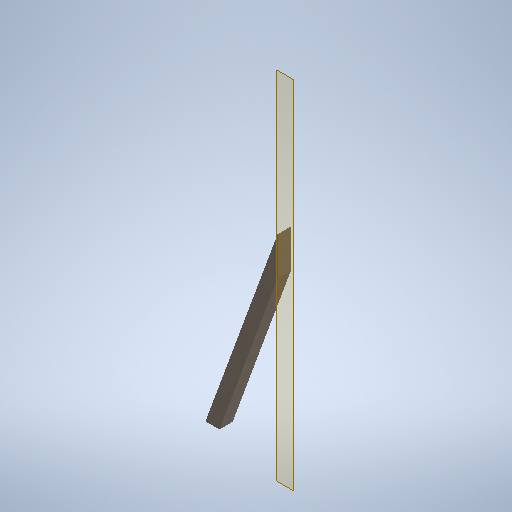
# Autodesk Inventor part: BaseAngularLarge
Saved by Autodesk Inventor 2025.2 (Build 292293000, 293)
## iProperties
Created: 2025-03-06
Part Number: BaseAngularLarge
Material: Wood (Walnut)
Document SubType Name: Modeling
Designer: baolo
Density: 0.55 g/cm^3
Appearance: Walnut
Mass: 84.4562 g
Surface Area: 320.992 cm^2
Volume: 153.557 cm^3
Author: baolo
Autodesk Inventor part; units mm, degrees
ref_plane "YZ Plane" through (0, 0, 0) normal (1, 0, 0) x (0, 1, 0)
ref_plane "XZ Plane" through (0, 0, 0) normal (0, 1, 0) x (-1, 0, 0)
ref_plane "XY Plane" through (0, 0, 0) normal (0, 0, 1) x (1, 0, 0)
ref_plane "Work Plane1" through (0, 0, 0) normal (0, 0, 1) x (1, 0, 0)
sketch "Sketch1" plane through (0, 0, 0) normal (0, 0, 1) x (1, 0, 0)
  line L0 (-95.7656, 0) -> (-77.1824, 0)
  line L1 (-77.1824, 0) -> (0, 212.057)
  line L2 (0, 212.057) -> (0, 263.1139)
  line L3 (0, 263.1139) -> (-95.7656, 0)
  line L4 (-205, 0) -> (-205, -20) construction
  line L5 (0, 0) -> (0, 430) construction
  line L6 (-205, 0) -> (225, 0) construction
  line L7 (-55.0006, 112.001) -> (-38.5912, 106.0285) construction
  line L8 (0, 263.1139) -> (16.4094, 257.1414) construction
  line L9 (16.4094, 257.1414) -> (0, 212.057) construction
  line L10 (-95.7656, 0) -> (-79.3563, -5.9725) construction
  line L11 (-79.3563, -5.9725) -> (-77.1824, 0) construction
  line L12 (-115.95, -17.4625) -> (-115.95, 0) construction
  dimension "d0" = 70
  dimension "d4" = 280
  constraints: 20 end point, 4 perpendicular, 3 point on line, 2 equal length, 1 collinear, 1 horizontal, 1 midpoint, 1 parallel, 1 vertical, 2 other
  measures "d0" angle of L6 L1
  measures "d4" distance of L2.end L0.start
ref_plane "Work Plane2" through (0, 0, -20) normal (0, 0, -1) x (0, 1, 0)
ref_plane "Work Plane3" through (-125, -17.4625, -17.4625) normal (0, 0, -1) x (0, 1, 0)
extrude "Extrusion1" add sketch "Sketch1" against normal up to surface (17.4625 mm away)
body "Solid1"
